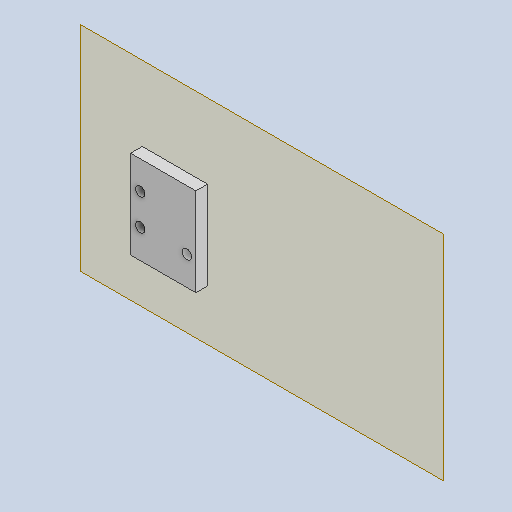
# Autodesk Inventor part: проставк
Saved by Autodesk Inventor 2024.2 (Build 282272000, 272)
## iProperties
Created: 2025-12-30
Part Number: проставк
Material: Типовые
Document SubType Name: Modeling
Designer: katya_notebook
Density: 1 g/cm^3
Appearance: По умолчанию
Author: katya_notebook
Autodesk Inventor part; units mm, degrees
ref_plane "YZ Plane" through (0, 0, 0) normal (1, 0, 0) x (0, 1, 0)
ref_plane "XZ Plane" through (0, 0, 0) normal (0, 1, 0) x (-1, 0, 0)
ref_plane "XY Plane" through (0, 0, 0) normal (0, 0, 1) x (1, 0, 0)
ref_plane "РабПлоскость1" through (51.8181, -3.2568, 14.8616) normal (0, 0, 1) x (1, 0, 0)
sketch "Эскиз1" plane through (51.8181, -3.2568, 14.8616) normal (0, 0, 1) x (1, 0, 0)
  circle A0 centre (-28.2721, 1.0327) radius 1.2 projected
  line L0 (-26.6721, 3.7827) -> (-26.6721, -9.7173)
  circle A1 centre (-28.2721, -6.9673) radius 0.8 projected
  circle A2 centre (-28.2721, -6.9673) radius 1.2 projected
  circle A3 centre (-16.2721, -6.9673) radius 1.2 projected
  line L1 (-29.8938, -55.4673) -> (-29.8938, 4.5327) projected
  line L2 (-30.7721, -9.7173) -> (-30.7721, -13.3173) projected
  line L3 (-13.9721, -9.7173) -> (-13.9721, 3.7827) projected
  line L4 (-30.7721, 8.2755) -> (-13.9721, 8.2755)
  line L5 (-13.9721, 8.2755) -> (-13.9721, -14.4178)
  line L6 (-13.9721, -14.4178) -> (-30.7721, -14.4178)
  line L7 (-30.7721, -14.4178) -> (-30.7721, 8.2755)
  circle A4 centre (-16.2721, 1.0327) radius 1.2 projected
  point P0 (-51.8181, 3.2568)
  point P1 (-30.7721, -9.7173)
  point P2 (-30.7721, -13.3173)
  point P3 (-13.9721, -9.7173)
  point P4 (-13.9721, 3.7827)
  point P5 (-15.1183, 0.7032)
  point P6 (-17.3217, 1.6144)
  constraints: 10 end point, 2 parallel, 1 horizontal, 1 perpendicular, 1 vertical, 2 other
extrude "Выдавливание1" add sketch "Эскиз1" along normal blind 3 contours L7 L4 L5 L3 L6 L2 | A4
